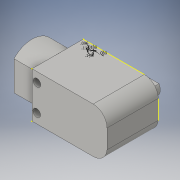
# Autodesk Inventor part: motor sumo jeffrey p
Saved by Autodesk Inventor 2016 (Build 200138000, 138)
## iProperties
Created: 2017-08-31
Part Number: motor sumo jeffrey p
Material: Generic
Document SubType Name: Modeling
Designer: student
Density: 1 g/cm^3
Appearance: Default
Author: student
Autodesk Inventor part; units mm, degrees
ref_plane "YZ Plane" through (0, 0, 0) normal (1, 0, 0) x (0, 1, 0)
ref_plane "XZ Plane" through (0, 0, 0) normal (0, 1, 0) x (-1, 0, 0)
ref_plane "XY Plane" through (0, 0, 0) normal (0, 0, 1) x (1, 0, 0)
sketch "Sketch1" plane through (0, 0, 0) normal (0, 0, 1) x (1, 0, 0)
  line L0 (-18.0458, -12.2355) -> (12.3135, -12.2355)
  line L1 (19.1466, -5.9617) -> (19.1466, 3.4363)
  line L2 (12.2886, 10.2943) -> (-18.0458, 10.2943)
  line L3 (-18.0458, 10.2943) -> (-18.0458, -12.2355)
  line L4 (-18.0458, -12.2355) -> (16.3456, 11.0826) construction
  line L5 (18.0458, -10.2943) -> (-18.0458, 10.2943) construction
  arc A0 (19.1466, 3.4363) -> (12.2886, 10.2943) centre (12.2886, 3.4363) ccw
  arc A1 (12.3135, -12.2355) -> (19.1466, -5.9617) centre (12.3135, -5.3775) ccw
  point P0 (0, 0)
  point P1 (19.1466, -1.2627)
  dimension "d3" = 22.5298
  dimension "d10" = 9.398
  dimension "d11" = 6.858
  dimension "d12" = 6.858
  constraints: 12 end point, 4 point on circle, 3 tangent, 2 centre point, 2 midpoint, 1 horizontal, 1 parallel, 1 point on line
  measures "d3" distance of L2.end L0.start
  measures "d10" distance of L1.start L1.end
  measures "d11" radius of A0
  measures "d12" radius of A1
extrude "Extrusion1" add sketch "Sketch1" along normal blind 25.4
sketch "Sketch2" plane through (0, 0, 0) normal (0, 0, -1) x (-1, 0, 0)
  line L0 (-12.2886, 10.2943) -> (18.0458, 10.2943) projected
  line L1 (18.0458, 10.2943) -> (18.0458, -12.2355) projected
  circle A0 centre (15.6074, 5.5191) radius 1.8796
  circle A1 centre (12.7451, 8.0337) radius 1.4732
  line L2 (-19.1466, -5.9617) -> (-19.1466, 3.4363) projected
  line L3 (18.0458, 10.2943) -> (18.0458, -12.2355) projected
  circle A2 centre (15.7097, -7.4978) radius 1.8796
  circle A3 centre (12.8872, -10.057) radius 1.4732
  point P0 (0, 0)
  dimension "d13" = 2.4384
  dimension "d14" = 4.7752
  dimension "d15" = 3.7592
  dimension "d16" = 2.9464
  dimension "d17" = 0.4572
  dimension "d18" = 2.2606
  constraints: 4 centre point
  measures "d13" distance from line of L1 A0.centre
  measures "d14" distance from line of L0 A0.centre
  measures "d15" diameter of A0
  measures "d16" diameter of A1
  measures "d18" distance from line of L0 A1.centre
sketch "Sketch3" plane through (0, 0, 0) normal (0, 0, -1) x (-1, 0, 0)
  circle A0 centre (-9.0374, 0) radius 4.445
  line L0 (-19.1466, -5.9617) -> (-19.1466, 3.4363) projected
  line L1 (-6.1855, -2.3622) -> (-11.9313, -2.3622)
  line L2 (-6.1855, 2.3622) -> (-11.9313, 2.3622)
  arc A1 (-6.1855, -2.3622) -> (-6.1855, 2.3622) centre (-10.1887, 0) ccw
  arc A2 (-11.9313, 2.3622) -> (-11.9313, -2.3622) centre (-7.9281, 0) ccw
  line L3 (-5.5405, 0) -> (-12.5763, 0)
  line L4 (-9.0584, 2.3622) -> (-9.0584, -2.3622)
  point P0 (0, 0)
  dimension "d23" = 8.89
  dimension "d24" = 10.1092
  dimension "d45" = 4.7244
  dimension "d46" = 4.6482
  dimension "d47" = 4.6482
  dimension "d48" = 7.0358
  constraints: 8 end point, 6 point on circle, 3 centre point, 2 horizontal, 2 midpoint
  measures "d23" diameter of A0
  measures "d24" distance from line of L0 A0.centre
  measures "d45" distance between parallel lines of L2 L1
  measures "d46" radius of A1
  measures "d47" radius of A2
sketch "Sketch4" plane through (-18.0458, -12.2355, 0) normal (-1, 0, 0) x (0, 0, 1)
  point P0 (0, 0)
  point P1 (25.4, 0)
  point P2 (0, 22.5298)
  point P3 (25.4, 22.5298)
extrude "Extrusion5" cut sketch "Sketch2" against normal blind 25.4 contours A2
extrude "Extrusion6" cut sketch "Sketch2" against normal blind 25.4 contours A0
extrude "Extrusion7" cut sketch "Sketch2" against normal blind 12.7 contours A1 | A3
sketch "Sketch5" plane through (-18.0458, -12.2355, 0) normal (-1, 0, 0) x (0, 0, 1)
  line L0 (25.4, 6.2738) -> (25.4, 15.6718) projected
  line L1 (0, 6.2738) -> (0, 15.6718) projected
  line L2 (0, 0) -> (25.4, 0) projected
  line L3 (12.7, 0) -> (12.7, 22.5298)
  line L4 (0, 22.5298) -> (25.4, 22.5298) projected
  line L5 (25.4, 0) -> (0, 22.5298)
  line L6 (25.4, 15.6718) -> (25.4, 22.5298) projected
  line L7 (0, 0) -> (25.4, 22.5298)
  line L8 (12.7, 3.937) -> (12.7, 18.5928) construction
  line L9 (21.6408, 3.937) -> (21.6408, 18.5928)
  line L10 (3.7592, 18.5928) -> (3.7592, 3.937)
  arc A0 (3.7592, 3.937) -> (21.6408, 3.937) centre (12.7, 12.1206) ccw
  arc A1 (21.6408, 18.5928) -> (3.7592, 18.5928) centre (12.7, 10.4092) ccw
  point P0 (0, 12.2355)
  point P1 (12.7, 11.2649)
  dimension "d39" = 22.5298
  dimension "d41" = 3.7592
  constraints: 14 end point, 6 point on circle, 4 midpoint, 2 centre point, 1 parallel, 1 point on line
  measures "d39" distance between parallel lines of L4 L2
  measures "d41" distance between parallel lines of L1 L10
extrude "Extrusion8" add sketch "Sketch5" along normal blind 12.7 contours A0 L7 L3 | L3 L5 A0 | A0 L10 A1 L5 L7 | L5 A1 L3 | L7 A1 L9 A0 L5 | L3 A1 L7
extrude "Extrusion9" add sketch "Sketch3" along normal blind 7.62 contours L1 L4 L3 A1 | L1 A2 L3 L4 | L3 L4 L2 A1 | L3 A2 L2 L4
body "Solid1"
